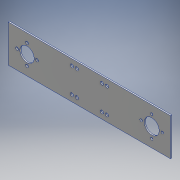
# Autodesk Inventor part: UpperArm1
Saved by Autodesk Inventor 2016 (Build 200138000, 138)
## iProperties
Created: 2016-06-25
Part Number: UpperArm1
Material: アルミニウム 6061
Document SubType Name: Modeling
Designer: 宏太
Density: 2.7 g/cm^3
Appearance: アルミニウム - フラット
Mass: 312.084 g
Surface Area: 370.98 cm^2
Volume: 115.587 cm^3
Author: 宏太
Autodesk Inventor part; units mm, degrees
ref_plane "YZ Plane" through (0, 0, 0) normal (1, 0, 0) x (0, 1, 0)
ref_plane "XZ Plane" through (0, 0, 0) normal (0, 1, 0) x (-1, 0, 0)
ref_plane "XY Plane" through (0, 0, 0) normal (0, 0, 1) x (1, 0, 0)
sketch "スケッチ1" plane through (0, 0, 0) normal (0, 1, 0) x (-1, 0, 0)
  line L0 (0, 0) -> (260, 0)
  line L1 (260, 0) -> (260, 60)
  line L2 (260, 60) -> (0, 60)
  line L3 (0, 60) -> (0, 0)
  dimension "d0" = 260
  dimension "d1" = 60
  constraints: 8 end point, 2 parallel, 1 horizontal, 1 perpendicular
  measures "d0" distance of L2.end L1.end
  measures "d1" distance of L1.end L0.end
extrude "押し出し1" add sketch "スケッチ1" along normal blind 2
sketch "スケッチ2" plane through (0, 0, 0) normal (0, 1, 0) x (-1, 0, 0)
  circle A0 centre (30, 30) radius 12
  line L0 (0, 60) -> (0, 0) projected
  line L1 (0, 0) -> (260, 0) projected
  dimension "d4" = 24
  dimension "d5" = 30
  dimension "d6" = 30
  constraints: 1 centre point
  measures "d4" diameter of A0
  measures "d5" distance from line of L0 A0.centre
  measures "d6" distance from line of L1 A0.centre
extrude "押し出し2" cut sketch "スケッチ2" along normal blind 10
sketch "スケッチ3" plane through (0, 2, 0) normal (0, 1, 0) x (1, 0, 0)
  circle A0 centre (-30, -30) radius 12 projected
  circle A1 centre (-30, -13) radius 2
  circle A2 centre (-13, -30) radius 2
  circle A3 centre (-47, -30) radius 2
  circle A4 centre (-30, -47) radius 2
  point P0 (0, 0)
  dimension "d10" = 4
  dimension "d11" = 4
  dimension "d12" = 4
  dimension "d13" = 4
  constraints: 4 centre point
  measures "d10" diameter of A1
  measures "d11" diameter of A2
  measures "d12" diameter of A3
  measures "d13" diameter of A4
extrude "押し出し3" cut sketch "スケッチ3" against normal blind 10 contours A1 | A2 | A3 | A4
sketch "スケッチ4" plane through (0, 0, 0) normal (0, -1, 0) x (1, 0, 0)
  circle A0 centre (-230, 30) radius 11.5
  line L0 (-260, 0) -> (-260, 60) projected
  point P0 (0, 0)
  dimension "d16" = 23
  dimension "d26" = 30
  constraints: 1 centre point
  measures "d16" diameter of A0
  measures "d26" distance from line of L0 A0.centre
extrude "押し出し4" cut sketch "スケッチ4" against normal blind 10
sketch "スケッチ5" plane through (0, 0, 0) normal (0, -1, 0) x (1, 0, 0)
  circle A0 centre (-230, 30) radius 11.5 projected
  circle A1 centre (-246, 30) radius 2.25
  circle A2 centre (-230, 46) radius 2.25
  circle A3 centre (-214, 30) radius 2.25
  circle A4 centre (-230, 14) radius 2.25
  point P0 (0, 0)
  dimension "d28" = 4.5
  dimension "d29" = 4.5
  dimension "d30" = 4.5
  dimension "d31" = 4.5
  constraints: 4 centre point
  measures "d28" diameter of A1
  measures "d29" diameter of A2
  measures "d30" diameter of A3
  measures "d31" diameter of A4
extrude "押し出し6" cut sketch "スケッチ5" against normal blind 10 contours A1 | A2 | A3 | A4
sketch "スケッチ6" plane through (0, 0, 0) normal (0, -1, 0) x (1, 0, 0)
  circle A0 centre (-158, 10) radius 2.6
  line L0 (0, 0) -> (-260, 0) projected
  circle A1 centre (-150, 10) radius 2.6
  circle A2 centre (-110, 10) radius 2.6
  circle A3 centre (-102, 10) radius 2.6
  circle A4 centre (-158, 50) radius 2.6
  line L1 (-260, 60) -> (0, 60) projected
  circle A5 centre (-150, 50) radius 2.6
  circle A6 centre (-110, 50) radius 2.6
  circle A7 centre (-102, 50) radius 2.6
  line L2 (-260, 0) -> (-260, 60) projected
  dimension "d34" = 5.2
  dimension "d35" = 10
  dimension "d36" = 5.2
  dimension "d37" = 8
  dimension "d38" = 5.2
  dimension "d39" = 40
  dimension "d40" = 5.2
  dimension "d41" = 8
  dimension "d42" = 5.2
  dimension "d43" = 10
  dimension "d44" = 5.2
  dimension "d45" = 5.2
  dimension "d46" = 5.2
  dimension "d49" = 102
  dimension "d50" = 40
  dimension "d51" = 8
  dimension "d52" = 8
  dimension "d53" = 102
  constraints: 8 centre point
  measures "d34" diameter of A0
  measures "d35" distance from line of L0 A0.centre
  measures "d36" diameter of A1
  measures "d37" distance of A1.centre A0.centre
  measures "d38" diameter of A2
  measures "d39" distance of A2.centre A1.centre
  measures "d40" diameter of A3
  measures "d41" distance of A3.centre A2.centre
  measures "d42" diameter of A4
  measures "d43" distance from line of L1 A4.centre
  measures "d44" diameter of A5
  measures "d45" diameter of A6
  measures "d46" diameter of A7
  measures "d49" distance from line of L2 A0.centre
  measures "d50" distance of A6.centre A5.centre
  measures "d51" distance of A7.centre A6.centre
  measures "d52" distance of A5.centre A4.centre
  measures "d53" distance from line of L2 A4.centre
extrude "押し出し7" cut sketch "スケッチ6" against normal blind 10
